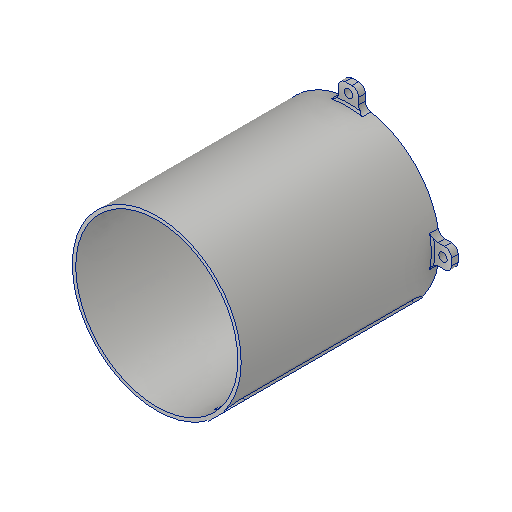
# Autodesk Inventor part: CNCM_ALU_Regolith_container
Saved by Autodesk Inventor 2025 (Build 290162010, 162A)
## iProperties
Created: 2018-09-12
Part Number: CNCM_ALU_Regolith_container
Material: Aluminum 6061
Document SubType Name: Modeling
Designer: Andrzej
Density: 2.7 g/cm^3
Appearance: Aluminum - Flat
Mass: 32.3159 g
Surface Area: 219.903 cm^2
Volume: 11.9688 cm^3
Author: Andrzej
Autodesk Inventor part; units mm, degrees
ref_plane "YZ Plane" through (0, 0, 0) normal (1, 0, 0) x (0, 1, 0)
ref_plane "XZ Plane" through (0, 0, 0) normal (0, 1, 0) x (-1, 0, 0)
sketch "Sketch1" plane through (0, 0, 0) normal (0, 0, 1) x (1, 0, 0)
  circle A0 centre (0, 0) radius 24
  circle A1 centre (0, 0) radius 25
  dimension "d0" = 48
  dimension "d1" = 1
  constraints: 2 centre point, 1 coincident
  measures "d0" diameter of A0
  measures "d1" radial gap between concentric circles of A0 A1
extrude "Extrusion1" add sketch "Sketch1" against normal blind 1.5 contours A0 | A1
extrude "Extrusion2" add sketch "Sketch1" along normal blind 57.3
chamfer "Chamfer1" distance 0.5 angle 45 1 edges at (-24, 0, 0)
sketch "Sketch2" plane through (0, 0, -1.5) normal (0, 0, -1) x (-1, 0, 0)
  circle A0 centre (0, 0) radius 25 projected
  circle A1 centre (0, 0) radius 25 projected
  line L0 (-3, 24.8193) -> (-3, 30.5)
  line L1 (-3, 30.5) -> (3, 30.5)
  line L2 (3, 30.5) -> (3, 24.8193)
  circle A2 centre (0, 28) radius 1.25
  dimension "d9" = 5.5
  dimension "d10" = 6
  dimension "d11" = 3
  dimension "d14" = 2.5
  dimension "d15" = 2.5
  constraints: 6 end point, 2 perpendicular, 2 point on circle, 1 centre point, 1 vertical
  measures "d9" distance edge to line of A0 L1
  measures "d10" distance between parallel lines of L2 L0
  measures "d11" distance from line of point (0, 0) L0
  measures "d14" diameter of A2
  measures "d15" distance from line of L1 A2.centre
extrude "Extrusion3" add sketch "Sketch2" against normal blind 2 contours A0 L0 L1 L2
fillet "Fillet1" radius 2 4 edges at (-3, 24.8193, -0.5) (3, 24.8193, -0.5) (3, 30.5, -0.5) (-3, 30.5, -0.5)
chamfer "Chamfer2" distance 0.5 angle 45 3 edges at (3.8169, 24.7069, 0.5) (0, 25, 0.5) (-3.8169, 24.7069, 0.5)
pattern_circular "Circular Pattern1" count 4 over 360 about axis through (0, 0, 0) along (0, 0, -1) of "Extrusion3", "Fillet1", "Chamfer2"
ref_plane "Work Plane1" through (17.6777, -17.6777, -1.5) normal (0.7071068, -0.7071068, 0) x (0.7071068, 0.7071068, 0)
sketch "Sketch3" plane through (17.6777, -17.6777, -1.5) normal (0.7071068, -0.7071068, 0) x (0.7071068, 0.7071068, 0)
  line L0 (0, 54.4) -> (0, 4.4) construction
  line L1 (-1.5, 54.4) -> (-1.5, 4.4)
  line L2 (1.5, 4.4) -> (1.5, 54.4)
  arc A0 (1.5, 54.4) -> (-1.5, 54.4) centre (0, 54.4) ccw
  arc A1 (-1.5, 4.4) -> (1.5, 4.4) centre (0, 4.4) ccw
  line L3 (-20.6456, 0) -> (-20.6456, 2.5) projected
  line L4 (-20.6456, 0) -> (-20.6456, 0) projected
  line L5 (-20.6456, 2.5) -> (-20.6456, 0) projected
  line L6 (-14.0983, 2.5) -> (-20.6456, 2.5) projected
  line L7 (-14.0983, 0) -> (-14.0983, 2.5) projected
  line L8 (14.0983, 0) -> (-14.0983, 0) projected
  line L9 (14.0983, 2.5) -> (14.0983, 0) projected
  line L10 (20.6456, 2.5) -> (14.0983, 2.5) projected
  line L11 (20.6456, 0) -> (20.6456, 2.5) projected
  line L12 (20.6456, 0) -> (20.6456, 0) projected
  line L13 (20.6456, 2.5) -> (20.6456, 0) projected
  line L14 (14.0983, 2.5) -> (20.6456, 2.5) projected
  line L15 (14.0983, 0) -> (14.0983, 2.5) projected
  line L16 (-14.0983, 0) -> (14.0983, 0) projected
  line L17 (-14.0983, 2.5) -> (-14.0983, 0) projected
  line L18 (-20.6456, 2.5) -> (-14.0983, 2.5) projected
  line L19 (25, 58.8) -> (-25, 58.8) projected
  line L20 (-5.6, 4.4) -> (-5.6, 54.4)
  line L21 (5.6, 54.4) -> (5.6, 4.4)
  line L22 (-4.1, 4.4) -> (-4.1, 54.4)
  arc A2 (4.1, 54.4) -> (-4.1, 54.4) centre (0, 54.4) ccw
  line L23 (4.1, 54.4) -> (4.1, 4.4)
  arc A3 (-4.1, 4.4) -> (4.1, 4.4) centre (0, 4.4) ccw
  line L24 (-2.5, 4.4) -> (-2.5, 54.4)
  arc A4 (2.5, 54.4) -> (-2.5, 54.4) centre (0, 54.4) ccw
  line L25 (2.5, 54.4) -> (2.5, 4.4)
  arc A5 (-2.5, 4.4) -> (2.5, 4.4) centre (0, 4.4) ccw
  arc A6 (5.6, 54.4) -> (3.4641, 58.8) centre (0, 54.4) ccw
  arc A7 (-3.4641, 58.8) -> (-5.6, 54.4) centre (0, 54.4) ccw
  arc A8 (-5.6, 4.4) -> (-3.4641, 0) centre (0, 4.4) ccw
  arc A9 (3.4641, 0) -> (5.6, 4.4) centre (0, 4.4) ccw
  point P0 (0, 1.5)
  point P1 (0, 29.4)
  point P2 (4.1, 29.4)
  point P3 (-4.1, 29.4)
  dimension "d23" = 3
  dimension "d24" = 50
  dimension "d25" = 25
  dimension "d26" = 50
  dimension "d27" = 58.8
  dimension "d28" = 4.1
  dimension "d29" = 2.6
  dimension "d30" = 1
  dimension "d31" = 4.4
  constraints: 20 end point, 20 point on circle, 10 centre point, 4 coincident, 4 parallel, 4 point on line, 4 tangent, 3 midpoint, 1 vertical, 6 other
  measures "d23" diameter of A1
  measures "d24" distance of L0.start L0.end
  measures "d25" distance from line of L0 L19.start
  measures "d26" distance of L19.start L19.end
  measures "d27" distance between parallel lines of L8 L19
  measures "d28" distance between parallel lines of L1 L20
  measures "d29" distance between parallel lines of L1 L22
  measures "d30" distance between parallel lines of L1 L24
  measures "d31" distance from line of L19 L0.start
extrude "Extrusion4" cut sketch "Sketch3" against normal blind 10 contours A0 L2 A1 L1
extrude "Extrusion5" add sketch "Sketch3" against normal blind 1 contours L8 A8 L20 A7 L19 A6 L21 A9 | L22 A2 L23 A3 | L24 A4 L25 A5
hole "Hole1" at (14.7785, -20.5768, 2.9) at (20.5768, -14.7785, 2.9) at (20.5768, -14.7785, 52.9) at (14.7785, -20.5768, 52.9) at (20.5768, -14.7785, 27.9) at (14.7785, -20.5768, 27.9) direction (-0.7071068, 0.7071068, 0) diameter 1.6 depth 8 tip angle 118
equation "\"d11\" = 0.5 * d10"
equation "\"d31\" = -0.5 * d24 + 0.5 * d27"
body "Solid1"
